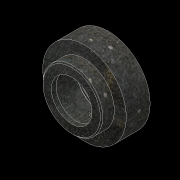
# Autodesk Inventor part: KON_Nietmaschine_Deckel
Saved by Autodesk Inventor 2019 (Build 230136000, 136)
## iProperties
Created: 2022-01-03
Part Number: KON_Nietmaschine_Deckel
Material: Stahl
Document SubType Name: Modeling
Designer: Jonas Nebl
Density: 7.85 g/cm^3
Appearance: Platte
Mass: 446.389 g
Surface Area: 165.843 cm^2
Volume: 56.8648 cm^3
Author: Jonas Nebl
Autodesk Inventor part; units mm, degrees
ref_plane "XZ Plane" through (0, 0, 0) normal (0, 1, 0) x (-1, 0, 0)
ref_plane "XY Plane" through (0, 0, 0) normal (0, 0, 1) x (1, 0, 0)
sketch "Skizze1" plane through (0, 0, 0) normal (0, 1, 0) x (-1, 0, 0)
  line L0 (17, 30.75) -> (17, 26.75)
  line L1 (17, 26.75) -> (20, 26.75)
  line L2 (20, 26.75) -> (20, 6.75)
  line L3 (23, 0) -> (35, 0)
  line L4 (35, 0) -> (35, 20)
  line L5 (35, 20) -> (25, 20)
  line L6 (25, 20) -> (25, 30.75)
  line L7 (17, 30.75) -> (25, 30.75)
  line L8 (0, 0) -> (0, 48.4152)
  line L9 (20, 6.75) -> (23, 6.75)
  line L10 (23, 6.75) -> (23, 4.75)
  line L11 (23, 4.75) -> (25, 4.75)
  line L12 (25, 4.75) -> (25, 3)
  line L13 (25, 3) -> (23, 3)
  line L14 (23, 3) -> (23, 0)
  point P0 (17, 4)
  dimension "d1" = 40
  dimension "d3" = 20
  dimension "d4" = 70
  dimension "d5" = 50
  dimension "d7" = 4
  dimension "d10" = 2
  dimension "d11" = 1.75
  dimension "d12" = 3
  dimension "d13" = 3
  dimension "d14" = 2
  dimension "d15" = 34
  dimension "d16" = 20
  constraints: 31 end point, 8 vertical, 7 horizontal, 3 point on line
  measures "d1" diameter of L2 L8
  measures "d3" distance of L3.end L4.end
  measures "d4" diameter of L4 L8
  measures "d5" diameter of L6 L8
  measures "d7" distance between parallel lines of L1 L7
  measures "d10" distance of L9.end L10.end
  measures "d11" distance of L11.end L12.end
  measures "d12" distance of L13.end L3.start
  measures "d13" distance of L2.end L9.end
  measures "d14" distance of L12.end L13.end
  measures "d15" diameter of L0 L8
  measures "d16" distance of L1.end L2.end
revolve "Umdrehung1" add sketch "Skizze1" angle 360 about axis through (0, 0, 0) along (0, 0, 1)
ref_plane "Arbeitsebene1" through (35, 0, 10) normal (1, 0, 0) x (0, 1, 0)
sketch "Skizze5" plane through (35, 0, 10) normal (1, 0, 0) x (0, 1, 0)
  line L0 (-36.029, 7.6022) -> (-33.5, 7.6022)
  line L1 (-33.5, 7.6022) -> (-33.5, -10.6796)
  line L2 (-33.5, -10.6796) -> (-36.029, -10.6796)
  line L3 (-36.029, -10.6796) -> (-36.029, 7.6022)
  line L4 (0, 27.0359) -> (0, -16.9655) projected
  point P0 (0, -10)
  dimension "d37" = 33.5
  constraints: 8 end point, 2 parallel, 1 horizontal, 1 perpendicular
  measures "d37" distance between parallel lines of L4 L1
extrude "Extrusion3" cut sketch "Skizze5" against normal through all
sketch "Skizze6" plane through (-10.1366, -33.5, 0) normal (0, -1, 0) x (1, 0, 0)
  line L0 (20.2731, 0) -> (0, 0) projected
  point P0 (10.1366, 0)
  point P1 (10.1366, 12)
  dimension "d47" = 12
  constraints: 1 vertical alignment
  measures "d47" distance from line of L0 point (10.137, 12)
hole "Bohrung2" at (0, -33.5, 12) direction (0, 1, 0) diameter 5 end up to face face through (0, 0, 16.75) facing (0, 0, -1) round with radius 20 far side no
thread "Gewinde1" size "M6x1" class "6H" standard "ANSI Metric M Profile" full length
chamfer "Fase2" distance 1 angle 45 1 edges at (25, 0, 30.75)
